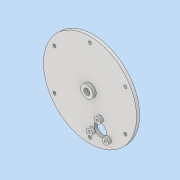
# Autodesk Inventor part: SpoolSectionSealingWall
Saved by Autodesk Inventor 2017 (Build 210142000, 142)
## iProperties
Created: 2016-11-06
Part Number: SpoolSectionSealingWall
Material: ABS Plastic
Document SubType Name: Modeling
Designer: techn
Density: 1.06 g/cm^3
Appearance: Smooth - White
Author: techn
Autodesk Inventor part; units mm, degrees
ref_plane "YZ Plane" through (0, 0, 0) normal (1, 0, 0) x (0, 1, 0)
ref_plane "XZ Plane" through (0, 0, 0) normal (0, 1, 0) x (-1, 0, 0)
ref_plane "XY Plane" through (0, 0, 0) normal (0, 0, 1) x (1, 0, 0)
sketch "Sketch1" plane through (0, 0, 0) normal (0, 0, 1) x (1, 0, 0)
  circle A0 centre (0, 0) radius 47.625
  dimension "d0" = 95.25
  constraints: 1 centre point, 1 coincident
  measures "d0" diameter of A0
extrude "Extrusion1" add sketch "Sketch1" along normal blind 3.175
sketch "Sketch2" plane through (0, 0, 3.175) normal (0, 0, 1) x (1, 0, 0)
  line L0 (0, 0) -> (0, 41.91)
  circle A0 centre (0, 41.91) radius 1.5875
  circle A1 centre (-36.2951, 20.955) radius 1.5875
  circle A2 centre (-36.2951, -20.955) radius 1.5875
  circle A3 centre (0, -41.91) radius 1.5875
  circle A4 centre (36.2951, -20.955) radius 1.5875
  circle A5 centre (36.2951, 20.955) radius 1.5875
  dimension "d3" = 41.91
  dimension "d4" = 3.175
  dimension "d7" = 360
  constraints: 6 centre point, 2 end point, 1 coincident, 1 vertical, 13 other
  measures "d3" distance of L0.start L0.end
  measures "d4" diameter of A0
extrude "Extrusion2" cut sketch "Sketch2" against normal blind 3.175
sketch "Sketch4" plane through (0, 0, 3.175) normal (0, 0, 1) x (1, 0, 0)
  circle A0 centre (10.541, -29.7561) radius 6.35
  point P0 (0, 0)
  dimension "d16" = 12.7
  dimension "d17" = 10.541
  dimension "d18" = 29.7561
  constraints: 1 centre point
  measures "d16" diameter of A0
  measures "d17" horizontal distance of A0.centre point (0, 0)
  measures "d18" vertical distance of A0.centre point (0, 0)
extrude "Extrusion4" cut sketch "Sketch4" against normal blind 3.175
sketch "Sketch5" plane through (0, 0, 3.175) normal (0, 0, 1) x (1, 0, 0)
  circle A0 centre (10.541, -29.7561) radius 6.35 projected
  line L0 (10.541, -29.7561) -> (10.541, -20.2311)
  circle A1 centre (10.541, -20.2311) radius 1.27
  circle A2 centre (10.541, -20.2311) radius 3.175
  circle A3 centre (2.2921, -34.5186) radius 3.175
  circle A4 centre (2.2921, -34.5186) radius 1.27
  circle A5 centre (18.7899, -34.5186) radius 3.175
  circle A6 centre (18.7899, -34.5186) radius 1.27
  point P0 (0, 0)
  dimension "d21" = 9.525
  dimension "d22" = 2.54
  dimension "d23" = 6.35
  dimension "d26" = 360
  constraints: 6 centre point, 4 coincident, 2 end point, 1 vertical, 13 other
  measures "d21" distance of L0.start L0.end
  measures "d22" diameter of A1
  measures "d23" diameter of A2
extrude "Extrusion5" add sketch "Sketch5" along normal blind 3.175 contours A5 | A3 | A2
extrude "Extrusion6" cut sketch "Sketch5" against normal blind 1.7145 contours A1 | A4 | A6
sketch "Sketch6" plane through (0, 0, 3.175) normal (0, 0, 1) x (1, 0, 0)
  circle A0 centre (0, 0) radius 3.175
  circle A1 centre (0, 0) radius 6.35
  dimension "d32" = 6.35
  dimension "d33" = 12.7
  dimension "d36" = 0
  dimension "d37" = 0
  constraints: 2 centre point, 1 coincident
  measures "d32" diameter of A0
  measures "d33" diameter of A1
  measures "d36" distance of point (0, 0) A0.centre
  measures "d37" distance of point (0, 0) A0.centre
extrude "Extrusion7" add sketch "Sketch6" along normal blind 3.175
body "Solid1"
